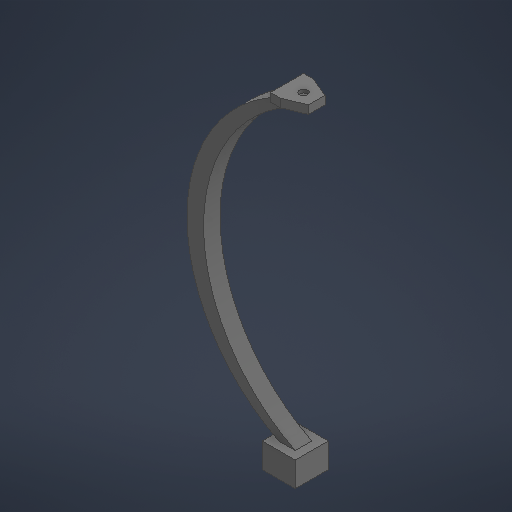
# Autodesk Inventor part: kakidrone
Saved by Autodesk Inventor 2026.1 (Build 301233000, 233)
## iProperties
Created: 2026-03-06
Part Number: kakidrone
Material: Generic
Document SubType Name: Modeling
Designer: ayjuni03
Density: 1 g/cm^3
Appearance: Default
Author: ayjuni03
Autodesk Inventor part; units mm, degrees
ref_plane "YZ Plane" through (0, 0, 0) normal (1, 0, 0) x (0, 1, 0)
ref_plane "XZ Plane" through (0, 0, 0) normal (0, 1, 0) x (-1, 0, 0)
ref_plane "XY Plane" through (0, 0, 0) normal (0, 0, 1) x (1, 0, 0)
sketch "Sketch1" plane through (0, 0, 0) normal (0, 0, 1) x (1, 0, 0)
  arc A0 (0, 0) -> (0, -180) centre (45.304, -90) ccw
  line L0 (-55.4554, -90) -> (-45.4554, -90) construction
  line L1 (0, -180) -> (0, -170) construction
  line L2 (0, 0) -> (0, -10) construction
  line L3 (0, -180) -> (10, -180) construction
  line L4 (0, 0) -> (10, 0) construction
  arc A1 (10, 0) -> (10, -180) centre (55.304, -90) ccw
  line L5 (0, 0) -> (10, 0)
  line L6 (10, -180) -> (0, -180)
  dimension "d0" = 180
  dimension "d1" = 10
  dimension "d2" = 10
  dimension "d3" = 10
  dimension "d4" = 10
  dimension "d5" = 10
  constraints: 14 end point, 6 point on circle, 4 horizontal, 2 centre point, 2 vertical, 1 collinear
  measures "d0" distance of L2.start L1.start
  measures "d1" distance of L0.start L0.end
  measures "d2" distance of L1.start L1.end
  measures "d3" distance of L2.start L2.end
  measures "d4" distance of L1.start L3.end
  measures "d5" distance of L2.start L4.end
extrude "Extrusion1" add sketch "Sketch1" along normal blind 10
sketch "Sketch2" plane through (0, 0, 0) normal (0, 1, 0) x (1, 0, 0)
  line L0 (-55.4554, -10) -> (0, -10) projected
  line L1 (0, -10) -> (0, -15)
  line L2 (0, -15) -> (0, 5)
  line L3 (0, 5) -> (6, 5)
  line L4 (0, -15) -> (6, -15)
  line L5 (6, -15) -> (18, -10)
  line L6 (6, 5) -> (18, 0)
  line L7 (18, 0) -> (18, -10)
  point P0 (0, 0)
  dimension "d8" = 5
  dimension "d9" = 20
  dimension "d10" = 6
  dimension "d11" = 13
  constraints: 14 end point, 1 horizontal, 1 perpendicular, 1 point on line, 1 vertical
  measures "d8" distance of L0.end L1.end
  measures "d9" distance of L1.end L2.end
  measures "d10" distance of L2.end L3.end
  measures "d11" distance of L4.end L5.end
extrude "Extrusion2" add sketch "Sketch2" along normal blind 5
sketch "Sketch3" plane through (0, -180, 0) normal (0, -1, 0) x (1, 0, 0)
  line L0 (0, -5) -> (0, 15) construction
  line L1 (0, 5) -> (-5, 5) construction
  line L2 (-5, 5) -> (0, 5) construction
  line L3 (0, 5) -> (-5, 5) construction
  line L4 (-5, 5) -> (-5, 15) construction
  line L5 (-5, 15) -> (15, 15) construction
  line L6 (15, 15) -> (15, -5) construction
  line L7 (15, -5) -> (-5, -5) construction
  line L8 (-5, -5) -> (-5, 5) construction
  line L9 (-5, 15) -> (15, 15)
  line L10 (15, -5) -> (-5, -5)
  line L11 (-5, 15) -> (-5, -5)
  line L12 (15, -5) -> (15, 15)
  point P0 (0, 0)
  dimension "d14" = 5
  dimension "d15" = 20
  dimension "d16" = 20
  constraints: 24 end point, 5 perpendicular, 3 collinear, 2 parallel, 1 horizontal, 1 midpoint, 1 point on line, 1 vertical
  measures "d14" distance of L1.start L1.end
  measures "d15" distance of L4.end L5.end
  measures "d16" distance of L5.end L6.end
extrude "Extrusion3" add sketch "Sketch3" along normal blind 15
sketch "Sketch4" plane through (0, 5, 0) normal (0, 1, 0) x (1, 0, 0)
  line L0 (10, 0) -> (10, -10) projected
  circle A0 centre (10, -5) radius 2.5
  point P0 (0, 0)
  dimension "d19" = 5
  constraints: 1 centre point, 1 midpoint
  measures "d19" diameter of A0
extrude "Extrusion4" cut sketch "Sketch4" against normal blind 2
body "Solid1"
